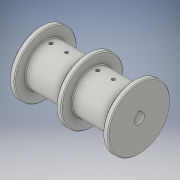
# Autodesk Inventor part: Drum
Saved by Autodesk Inventor 2016 (Build 200138000, 138)
## iProperties
Created: 2016-03-01
Part Number: Drum
Material: UHMW, White
Document SubType Name: Modeling
Designer: agmle
Mass: 973 g
Surface Area: 628.317 cm^2
Volume: 360.37 cm^3
Density: 0.94 g/cm^3
Appearance: Smooth - White
Author: agmle
Autodesk Inventor part; units mm, degrees
ref_plane "YZ Plane" through (0, 0, 0) normal (1, 0, 0) x (0, 1, 0)
ref_plane "XZ Plane" through (0, 0, 0) normal (0, 1, 0) x (-1, 0, 0)
ref_plane "XY Plane" through (0, 0, 0) normal (0, 0, 1) x (1, 0, 0)
sketch "Sketch1" plane through (0, 0, 0) normal (0, 1, 0) x (-1, 0, 0)
  line L0 (0, -12.7) -> (0, -38.1)
  line L1 (0, -38.1) -> (-6.35, -38.1)
  line L2 (-6.35, -38.1) -> (-6.35, -25.4)
  line L3 (-6.35, -25.4) -> (-57.15, -25.4)
  line L4 (-57.15, -25.4) -> (-57.15, -38.1)
  line L5 (-57.15, -38.1) -> (-63.5, -38.1)
  line L6 (-63.5, -38.1) -> (-63.5, -25.4)
  line L7 (-63.5, -25.4) -> (-114.3, -25.4)
  line L8 (-114.3, -25.4) -> (-114.3, -38.1)
  line L9 (-114.3, -38.1) -> (-120.65, -38.1)
  line L10 (-120.65, -38.1) -> (-120.65, 0)
  line L11 (-120.65, 0) -> (-3.175, 0)
  line L12 (0, -12.7) -> (-3.175, -12.7)
  line L13 (-3.175, -12.7) -> (-3.175, 0)
  line L14 (-3.175, 0) -> (0, 0) construction
  line L15 (0, 0) -> (0, -12.7) construction
  dimension "d1" = 25.4
  dimension "d2" = 6.35
  dimension "d3" = 50.8
  dimension "d52" = 38.1
  dimension "d53" = 3.175
  dimension "d54" = 12.7
  constraints: 32 end point, 9 perpendicular, 7 point on line, 3 collinear, 3 horizontal, 1 coincident, 1 vertical
  measures "d1" distance between parallel lines of L11 L3
  measures "d2" distance of L0.end L1.end
  measures "d3" distance of L2.end L3.end
  measures "d52" distance between parallel lines of L11 L1
  measures "d53" distance between parallel lines of L0 L13
  measures "d54" distance between parallel lines of L12 L11
revolve "Revolution1" add sketch "Sketch1" angle 360 about axis through (120.65, 0, 0) along (-1, 0, 0)
hole "Hole1" at (120.65, 0, 0) direction (-1, 0, 0) diameter 12.7 end through all
chamfer "Chamfer1" distance 1 angle 45 10 edges at (6.35, 0, 38.1) (0, 0, 38.1) (6.35, 0, 25.4) (57.15, 0, 38.1) (63.5, 0, 38.1) (57.15, 0, 25.4) (63.5, 0, 25.4) (114.3, 0, 38.1) (120.65, 0, 38.1) (114.3, 0, 25.4)
sketch "Sketch2" plane through (120.65, 0, 0) normal (1, 0, 0) x (0, 0, -1)
  line L0 (-1.5875, 7.9375) -> (1.5875, 7.9375)
  line L1 (1.5875, 7.9375) -> (1.5875, 4.7625)
  line L2 (1.5875, 4.7625) -> (-1.5875, 4.7625)
  line L3 (-1.5875, 4.7625) -> (-1.5875, 7.9375)
  circle A0 centre (0, 0) radius 6.35 construction
  line L4 (-1.5875, 6.35) -> (1.5875, 6.35) construction
  point P0 (0, 6.35)
  dimension "d21" = 3.175
  dimension "d22" = 3.175
  constraints: 10 end point, 3 midpoint, 2 horizontal, 2 parallel, 1 perpendicular, 1 vertical alignment, 1 other
  measures "d21" distance of L2.end L0.start
  measures "d22" distance of L0.start L0.end
extrude "Extrusion1" cut sketch "Sketch2" against normal through all
ref_plane "Work Plane1" through (88.9, 25.4, 0) normal (0, -1, 0) x (1, 0, 0)
sketch "Sketch3" plane through (88.9, 25.4, 0) normal (0, -1, 0) x (1, 0, 0)
  line L0 (-81.55, 25.4) -> (-32.75, 25.4) construction
  line L1 (-82.55, 37.1) -> (-82.55, -37.1) construction
  line L2 (-81.55, -25.4) -> (-32.75, -25.4) construction
  line L3 (-31.75, -37.1) -> (-31.75, 37.1) construction
  line L4 (-25.4, 37.1) -> (-25.4, -37.1) construction
  line L5 (-24.4, -25.4) -> (24.4, -25.4) construction
  line L6 (-24.4, 25.4) -> (24.4, 25.4) construction
  line L7 (25.4, -37.1) -> (25.4, 37.1) construction
  line L8 (-57.15, 25.4) -> (-57.15, -25.4) construction
  line L9 (0, -25.4) -> (0, 25.4) construction
  point P0 (-88.9, 0)
  point P1 (-57.15, 0)
  point P2 (0, 0)
  constraints: 6 midpoint, 4 end point
hole "Hole2" at (31.75, 25.4, 0) at (88.9, 25.4, 0) direction (0, -1, 0) diameter 3.683 end up to surface thread size "10-24 UNC" class "2B" standard "ANSI Unified Screw Threads"
sketch "Sketch5" plane through (88.9, 25.4, 0) normal (0, -1, 0) x (1, 0, 0)
  line L0 (-57.15, -1.8415) -> (0, -1.8415) construction
  line L1 (0, 1.8415) -> (-57.15, 1.8415) construction
  line L2 (-55.3085, 1.8415) -> (-55.3085, -1.8415) construction
  line L3 (-1.8415, 1.8415) -> (-1.8415, -1.8415) construction
  line L4 (-1.8415, 0) -> (-55.3085, 0) construction
  line L5 (-55.3085, 0) -> (-76.2, 0) construction
  line L6 (-82.55, 37.1) -> (-82.55, -37.1) construction
  line L7 (-25.4, 37.1) -> (-25.4, -37.1) construction
  point P0 (-88.9, 0)
  point P1 (-19.05, 0)
  dimension "d43" = 6.35
  dimension "d44" = 6.35
  constraints: 12 end point, 5 point on line, 4 horizontal, 2 midpoint, 2 perpendicular, 2 vertical, 1 parallel, 8 other
  measures "d43" distance from line of L6 L5.end
  measures "d44" distance from line of L7 point (-19.05, 0)
hole "Hole4" at (12.7, 25.4, 0) at (69.85, 25.4, 0) direction (0, -1, 0) diameter 4.1402 depth 17.4625 tip angle 118
equation "\"d1\" = 0.5 * Drum_Spool_OD"
equation "\"d2\" = Drum_Wall_Width"
equation "\"d3\" = Drum_Spool_Width"
equation "\"d52\" = 0.5 * Drum_Wall_OD"
equation "\"d7\" = Gearbox_Shaft_OD"
equation "\"d18\" = Break_Edge"
equation "\"d21\" = Gearbox_Shaft_Key_Height"
equation "\"d22\" = Gearbox_Shaft_Key_Width"
equation "\"Gearbox_Shaft_OD\" = 12.7"
equation "\"Gearbox_Shaft_Key_Width\" = 3.175"
equation "\"Gearbox_Shaft_Key_Height\" = 3.175"
equation "\"Drum_Spool_OD\" = 50.8"
equation "\"Drum_Wall_OD\" = 76.2"
equation "\"Drum_Spool_Width\" = 50.8"
equation "\"Drum_Wall_Width\" = 6.35"
equation "\"Fitting_Break\" = 2"
equation "\"Break_Edge\" = 1"
body "Solid1"
